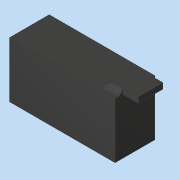
# Autodesk Inventor part: ASDSBattery
Saved by Autodesk Inventor 2018 (Build 220112000, 112)
## iProperties
Created: 2019-07-29
Part Number: ASDSBattery
Material: ABS Plastic
Document SubType Name: Modeling
Designer: Derek Wider
Density: 1.06 g/cm^3
Appearance: Smooth - Black
Author: Derek Wider
Autodesk Inventor part; units mm, degrees
ref_plane "YZ Plane" through (0, 0, 0) normal (1, 0, 0) x (0, 1, 0)
ref_plane "XZ Plane" through (0, 0, 0) normal (0, 1, 0) x (-1, 0, 0)
ref_plane "XY Plane" through (0, 0, 0) normal (0, 0, 1) x (1, 0, 0)
sketch "Sketch1" plane through (0, 0, 0) normal (0, 0, 1) x (1, 0, 0)
  line L0 (0, 0) -> (59.944, 0)
  line L1 (59.944, 0) -> (59.944, 31.496)
  line L2 (59.944, 31.496) -> (0, 31.496)
  line L3 (0, 31.496) -> (0, 0)
  dimension "d0" = 59.944
  dimension "d1" = 31.496
  constraints: 8 end point, 2 parallel, 1 horizontal, 1 perpendicular
  measures "d0" distance of L2.end L1.end
  measures "d1" distance of L1.end L0.end
extrude "Extrusion1" add sketch "Sketch1" along normal blind 22.606
sketch "Sketch2" plane through (59.944, 0, 0) normal (1, 0, 0) x (0, 0, -1)
  line L0 (-4.318, 31.496) -> (-18.288, 31.496)
  line L1 (-18.288, 31.496) -> (-18.288, 34.671)
  line L2 (-18.288, 34.671) -> (-4.318, 34.671)
  line L3 (-4.318, 34.671) -> (-4.318, 31.496)
  line L4 (0, 31.496) -> (-22.606, 31.496) projected
  point P0 (0, 0)
  point P1 (-11.303, 34.671)
  point P2 (-11.303, 31.496)
  point P3 (-11.303, 31.496)
  dimension "d4" = 13.97
  dimension "d5" = 3.175
  constraints: 8 end point, 3 midpoint, 2 parallel, 1 coincident, 1 horizontal, 1 perpendicular, 1 point on line, 1 vertical alignment
  measures "d4" distance of L1.end L2.end
  measures "d5" distance of L2.end L0.start
extrude "Extrusion2" add sketch "Sketch2" along normal blind 8.89 and the other way blind 6.35
fillet "Fillet1" radius 3.175 3 edges at (53.594, 31.496, 11.303) (56.769, 31.496, 18.288) (56.769, 31.496, 4.318)
body "Solid1"
